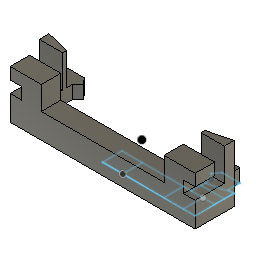
Celestron USB Cable Holder (Autodesk Fusion 360 design; units mm, degrees)
Autodesk Fusion 360 part; units mm, degrees
sketch "Sketch1" plane through (0, 0, 0) normal (0, 0, 1) x (1, 0, 0)
  line L0 (23.6957, -0.0182) -> (23.6957, -10.0069)
  line L1 (-0.0543, -10.0069) -> (23.6957, -10.0069)
  line L2 (17.7267, -0.0264) -> (17.7267, -5.0176)
  line L3 (-0.0543, -5.0176) -> (17.7267, -5.0176)
  line L4 (5.1457, -10.0069) -> (5.1457, -5.0176)
  line L5 (17.7267, -0.0264) -> (16.3734, 1.4275)
  line L6 (17.5959, 2.993) -> (16.3734, 1.4275)
  line L7 (23.6957, -0.0182) -> (22.197, -0.0182)
  line L8 (23.6957, -0.0182) -> (17.7267, -1.5064)
  line L9 (-0.0543, -5.0176) -> (-0.0543, -10.0069)
  line L10 (17.5959, 2.993) -> (22.197, 2.993)
  line L11 (22.197, -0.0182) -> (22.197, 2.993)
  line L12 (23.6957, -0.0182) -> (22.197, -0.0182) construction
  line L13 (17.7267, -5.0176) -> (23.6957, -5.0125)
  line L14 (15.6957, -5.0176) -> (15.6957, -10.0069)
  line L15 (20.6957, -5.0176) -> (20.6957, -10.0069)
  line L16 (17.7267, -2.522) -> (23.6957, -2.522)
  point P0 (17.7267, -0.0264)
  point P1 (5.1457, -10.0069)
  dimension "latch_width" = 5.969
  dimension "d8" = 5.2
  dimension "d16" = 14
  dimension "d26" = 3
  dimension "d27" = 5
  dimension "d41" = 23.75
  constraint coincident P0 L2.start
  constraint coincident L1 P1
  constraint coincident P1 L4.start
  constraint coincident L3 L4.end
  constraint perpendicular L0 L7
  constraint parallel L1 L3
  constraint horizontal L12
  constraint coincident L2 L8.end
  constraint coincident L3.start L9.start
  constraint coincident L1.start L9.end
  constraint perpendicular L1 L9
  constraint equal L5 L6
  constraint parallel L0 L9
  constraint parallel L1 L10
  constraint parallel L0 L11
  constraint parallel L0 L2
  constraint midpoint L0 L13.end
  constraint coincident L3 L14.start
  constraint coincident L1 L14.end
  constraint perpendicular L1 L14
  constraint coincident L1 L15.end
  constraint perpendicular L1 L15
  constraint midpoint L2 L16.start
  constraint coincident L0 L16.end
  constraint perpendicular L0 L16
  measures "latch_width" distance of L0.start P0
  measures "d8" distance of L1.start P1
  measures "d16" angle of L8 L12
  measures "d26" distance of L0 L15
  measures "d27" distance of L14 L15
  measures "d41" distance of L0 L9
extrude "Extrude4" add sketch "Sketch1" along normal blind 3.4 makes body 1
extrude "Extrude9" add sketch "Sketch1" against normal blind 3 contours L0 L2 L8 L16 | L0 L2 L13 L16 | L0 L1 L3 L13 L14 | L1 L3 L4 L14 | L1 L3 L4 L9 bodies 1
extrude "Extrude5" add sketch "Sketch1" along normal blind 11.7 contours L0 L2 L8 L16 bodies 1
extrude "Extrude6" add sketch "Sketch1" along normal blind 9.4 contours L0 L1 L3 L13 L14 bodies 1
sketch "Sketch2" plane through (23.6957, 0, 0) normal (1, 0, 0) x (0, 1, 0)
  line L0 (-0.0182, 0) -> (-0.0182, 3.4)
  line L1 (-0.0182, 3.4) -> (-0.0182, 11.7)
  line L2 (-0.0182, 11.7) -> (-2.522, 11.7)
  line L3 (-2.522, 11.7) -> (-2.522, 3.4)
  line L4 (-2.522, 3.4) -> (-5.0125, 3.4)
  line L5 (-5.0125, 3.4) -> (-5.0125, 9.4)
  line L6 (-5.0125, 9.4) -> (-10.0069, 9.4)
  line L7 (-10.0069, 9.4) -> (-10.0069, -3)
  line L8 (-5.0125, 3.4) -> (-10.0069, 3.4)
  line L9 (-10.0069, 3.4) -> (-10.0069, 6.4)
  line L10 (-10.0069, 6.4) -> (-5.0125, 6.4)
  line L11 (-5.0125, 6.4) -> (-5.0125, 3.4)
  line L12 (-10.0069, -3) -> (-0.0182, -3)
  line L13 (-0.0182, -3) -> (-0.0182, 0)
  dimension "d34" = 3
  constraint horizontal L8
  constraint vertical L9
  constraint horizontal L10
  constraint vertical L11
  constraint coincident L7 L9.end
  constraint coincident L4.end L5.start
  measures "d34" distance of L8.end L9.end
extrude "Extrude7" cut sketch "Sketch2" against normal blind 3 contours L5 L7 L8 L9 L10 L11 bodies 1
mirror "Mirror1" about plane through (-0.0543, -5.0176, 0) normal (-1, 0, 0) of bodies 1 makes body 2
extrude "Extrude8" add 1 faces at (-0.0543, -8.3438, 1.2667) along direction (-1, 0, 0) blind 2 on bodies 1 bodies 1 2
equation "usbconn_width = 10.4 mm"
equation "usbconn_height = 8.3 mm"
equation "d8 = usbconn_width / 2"
equation "slot_height = 3.4 mm"
equation "d28 = slot_height"
equation "d30 = slot_height + usbconn_height"
equation "d32 = slot_height + 6 mm"
equation "d41 = width"
equation "width = 23.75 mm"
